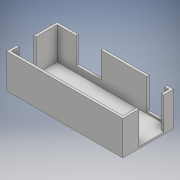
# Autodesk Inventor part: PlutoIIxHDMI
Saved by Autodesk Inventor 2018 (Build 220112000, 112)
## iProperties
Created: 2018-03-05
Part Number: PlutoIIxHDMI
Material: Generic
Document SubType Name: Modeling
Designer: matth
Density: 1 g/cm^3
Appearance: Default
Author: matth
Autodesk Inventor part; units mm, degrees
ref_plane "YZ Plane" through (0, 0, 0) normal (1, 0, 0) x (0, 1, 0)
ref_plane "XZ Plane" through (0, 0, 0) normal (0, 1, 0) x (-1, 0, 0)
ref_plane "XY Plane" through (0, 0, 0) normal (0, 0, 1) x (1, 0, 0)
sketch "Sketch1" plane through (0, 0, 0) normal (0, 0, 1) x (1, 0, 0)
  line L0 (-7.6232, 4.5478) -> (61.5768, 4.5478)
  line L1 (61.5768, 4.5478) -> (61.5768, -23.9522)
  line L2 (61.5768, -23.9522) -> (-7.6232, -23.9522)
  line L3 (-7.6232, -23.9522) -> (-7.6232, 4.5478)
  line L4 (62.9768, 5.9478) -> (-9.0232, 5.9478)
  line L5 (-9.0232, 5.9478) -> (-9.0232, -25.3522)
  line L6 (-9.0232, -25.3522) -> (62.9768, -25.3522)
  line L7 (62.9768, -25.3522) -> (62.9768, 5.9478)
  point P0 (0, 0)
  dimension "d0" = 69.2
  dimension "d1" = 28.5
  dimension "d2" = 1.4
  constraints: 16 end point, 4 parallel, 2 perpendicular, 1 horizontal, 3 other
  measures "d0" distance of L1.end L2.end
  measures "d1" distance of L0.end L1.end
  measures "d2" distance between parallel lines of L0 L4
extrude "Extrusion1" add sketch "Sketch1" along normal blind 20
sketch "Sketch2" plane through (0, 0, 0) normal (0, 0, -1) x (-1, 0, 0)
  line L0 (9.0232, 5.9478) -> (9.0232, -25.3522) projected
  line L1 (-62.9768, 5.9478) -> (9.0232, 5.9478) projected
  line L2 (9.0232, -25.3522) -> (-62.9768, -25.3522) projected
  line L3 (-62.9768, -25.3522) -> (-62.9768, 5.9478) projected
  point P0 (0, 0)
extrude "Extrusion2" add sketch "Sketch2" along normal blind 1.2
sketch "Sketch3" plane through (62.9768, -25.3522, 20) normal (1, 0, 0) x (0, 0, -1)
  line L0 (20, 29.9) -> (0, 29.9) projected
  line L1 (20, 1.4) -> (0, 1.4) projected
  line L2 (20, 1.4) -> (20, 29.9) projected
  line L3 (20, 25.4) -> (14, 25.4)
  line L4 (14, 25.4) -> (14, 9.9)
  line L5 (14, 9.9) -> (20, 9.9)
  line L6 (20, 9.9) -> (20, 25.4)
  point P0 (20, 25.3522)
  dimension "d7" = 4.5
  dimension "d8" = 6
  dimension "d9" = 15.5
  constraints: 8 end point, 2 parallel, 1 horizontal, 1 perpendicular, 1 point on line
  measures "d7" distance between parallel lines of L0 L3
  measures "d8" distance of L3.start L3.end
  measures "d9" distance of L3.end L4.end
extrude "Extrusion3" cut sketch "Sketch3" against normal up to surface (1.4 mm away)
sketch "Sketch4" plane through (-9.0232, 5.9478, 20) normal (0, 1, 0) x (1, 0, 0)
  line L0 (70.6, 20) -> (70.6, 0) projected
  line L1 (70.6, 20) -> (1.4, 20) projected
  line L2 (68, 18.9) -> (57, 18.9)
  line L3 (57, 18.9) -> (57, 13.5)
  line L4 (57, 13.5) -> (68, 13.5)
  line L5 (68, 13.5) -> (68, 18.9)
  point P0 (9.0232, 20)
  dimension "d12" = 11
  dimension "d13" = 2.6
  dimension "d14" = 1.1
  dimension "d15" = 5.4
  constraints: 8 end point, 2 parallel, 1 horizontal, 1 perpendicular
  measures "d12" distance of L3.end L4.end
  measures "d13" distance between parallel lines of L5 L0
  measures "d14" distance between parallel lines of L1 L2
  measures "d15" distance between parallel lines of L2 L4
extrude "Extrusion4" cut sketch "Sketch4" against normal up to surface (1.4 mm away)
chamfer "Chamfer1" distance 2 angle 45 1 edges at (62.2768, -15.4522, 6)
chamfer "Chamfer2" distance 2 angle 45 1 edges at (62.2768, 0.0478, 6)
sketch "Sketch5" plane through (-9.0232, 5.9478, 20) normal (0, 1, 0) x (1, 0, 0)
  line L0 (1.4, 20) -> (1.4, 0) projected
  line L1 (70.6, 20) -> (1.4, 20) projected
  line L2 (13.1, 16) -> (28.6, 16)
  line L3 (28.6, 16) -> (28.6, 9.8)
  line L4 (28.6, 9.8) -> (13.1, 9.8)
  line L5 (13.1, 9.8) -> (13.1, 16)
  point P0 (9.0232, 20)
  dimension "d24" = 4
  dimension "d25" = 6.2
  dimension "d26" = 15.5
  dimension "d27" = 11.7
  constraints: 8 end point, 2 parallel, 1 horizontal, 1 perpendicular
  measures "d24" distance between parallel lines of L1 L2
  measures "d25" distance between parallel lines of L4 L2
  measures "d26" distance of L3.end L4.end
  measures "d27" distance between parallel lines of L0 L5
extrude "Extrusion5" cut sketch "Sketch5" against normal up to surface (1.4 mm away)
chamfer "Chamfer3" distance 2 angle 45 2 edges at (4.0768, 5.2478, 10.2) (19.5768, 5.2478, 10.2)
sketch "Sketch6" plane through (-9.0232, -25.3522, 20) normal (-1, 0, 0) x (0, 0, 1)
  line L0 (-20, 1.4) -> (0, 1.4) projected
  line L1 (-20, 29.9) -> (-20, 1.4) projected
  line L2 (-14.8, 6.4) -> (-9.6, 6.4)
  line L3 (-9.6, 6.4) -> (-9.6, 16.9)
  line L4 (-9.6, 16.9) -> (-14.8, 16.9)
  line L5 (-14.8, 16.9) -> (-14.8, 6.4)
  point P0 (-20, 25.3522)
  dimension "d33" = 5
  dimension "d34" = 10.5
  dimension "d35" = 5.2
  dimension "d36" = 5.2
  constraints: 8 end point, 2 parallel, 1 horizontal, 1 perpendicular
  measures "d33" distance between parallel lines of L0 L2
  measures "d34" distance of L2.end L3.end
  measures "d35" distance of L2.start L2.end
  measures "d36" distance between parallel lines of L1 L5
extrude "Extrusion6" cut sketch "Sketch6" against normal up to surface (1.4 mm away)
sketch "Sketch8" plane through (62.9768, -25.3522, 20) normal (1, 0, 0) x (0, 0, -1)
  line L0 (16, 9.9) -> (20, 9.9) projected
  line L1 (0, 29.9) -> (0, 1.4) projected
  line L2 (16, 9.9) -> (0, 9.9)
  line L3 (0, 9.9) -> (0, 25.3522)
  line L4 (0, 25.3522) -> (16, 25.3522)
  line L5 (16, 25.3522) -> (16, 9.9)
  point P0 (20, 25.3522)
  constraints: 8 end point, 2 parallel, 1 horizontal, 1 perpendicular, 1 point on line
extrude "Extrusion7" cut sketch "Sketch8" against normal up to surface (1.4 mm away)
sketch "Sketch9" plane through (-7.6232, 4.5478, 20) normal (0, -1, 0) x (1, 0, 0)
  line L0 (27.2, -11.8) -> (25.2, -9.8) projected
  line L1 (13.7, -9.8) -> (11.7, -11.8) projected
  line L2 (0, 0) -> (69.2, 0) projected
  line L3 (11.7, -11.8) -> (27.2, -11.8)
  line L4 (27.2, -11.8) -> (27.2, 0)
  line L5 (27.2, 0) -> (11.7, 0)
  line L6 (11.7, 0) -> (11.7, -11.8)
  line L7 (55.6, -13.5) -> (66.6, -13.5) projected
  line L8 (55.6, -13.5) -> (66.6, -13.5)
  line L9 (66.6, -13.5) -> (66.6, 0)
  line L10 (66.6, 0) -> (55.6, 0)
  line L11 (55.6, 0) -> (55.6, -13.5)
  point P0 (7.6232, -20)
  constraints: 16 end point, 4 parallel, 2 horizontal, 2 perpendicular, 2 point on line
extrude "Extrusion8" cut sketch "Sketch9" against normal up to surface (1.4 mm away)
sketch "Sketch10" plane through (-9.0232, -25.3522, 20) normal (-1, 0, 0) x (0, 0, 1)
  line L0 (-9.6, 16.9) -> (-9.6, 6.4) projected
  line L1 (0, 1.4) -> (0, 29.9) projected
  line L2 (-9.6, 6.4) -> (0, 6.4)
  line L3 (0, 6.4) -> (0, 16.9)
  line L4 (0, 16.9) -> (-9.6, 16.9)
  line L5 (-9.6, 16.9) -> (-9.6, 6.4)
  point P0 (-20, 25.3522)
  constraints: 8 end point, 2 parallel, 1 horizontal, 1 perpendicular, 1 point on line
extrude "Extrusion9" cut sketch "Sketch10" against normal up to surface (1.4 mm away)
body "Solid1"
